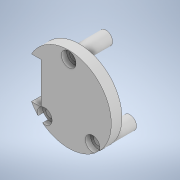
# Autodesk Inventor part: Driveunit_Spacer
Saved by Autodesk Inventor 2021 (Build 250183000, 183)
## iProperties
Created: 2024-08-04
Part Number: Driveunit_Spacer
Material: Generic
Document SubType Name: Modeling
Designer: Lukas
Density: 1 g/cm^3
Appearance: Default
Author: Lukas
Autodesk Inventor part; units mm, degrees
ref_plane "YZ Plane" through (0, 0, 0) normal (1, 0, 0) x (0, 1, 0)
ref_plane "XZ Plane" through (0, 0, 0) normal (0, 1, 0) x (-1, 0, 0)
ref_plane "XY Plane" through (0, 0, 0) normal (0, 0, 1) x (1, 0, 0)
sketch "Sketch1" plane through (0, 0, 0) normal (0, 0, 1) x (1, 0, 0)
  circle A0 centre (0, 0) radius 16
  line L0 (-16, 7.75) -> (-10.3, 7.75)
  line L1 (-10.3, 7.75) -> (-10.3, -7.75)
  line L2 (-10.3, -7.75) -> (-16, -7.75)
  line L3 (-16, -7.75) -> (-16, 7.75)
  circle A1 centre (-9, -10) radius 1.6
  circle A2 centre (9, -10) radius 1.6
  circle A3 centre (0, 13) radius 1.6
  circle A4 centre (0, 13) radius 2.5
  circle A5 centre (-9, -10) radius 2.5
  circle A6 centre (9, -10) radius 2.5
  point P0 (-10.3, 0)
  point P1 (-13.9978, -7.75)
  point P2 (-13.9978, 7.75)
  dimension "d0" = 32
  dimension "d1" = 5.7
  dimension "d2" = 15.5
  dimension "d3" = 9
  dimension "d4" = 9
  dimension "d5" = 23
  dimension "d6" = 13
  dimension "d7" = 3.2
  dimension "d8" = 5
  constraints: 8 end point, 7 centre point, 4 coincident, 4 equal radius, 2 horizontal alignment, 2 parallel, 1 horizontal, 1 midpoint, 1 perpendicular, 1 tangent, 1 vertical alignment
  measures "d0" diameter of A0
  measures "d1" distance of L0.start L0.end
  measures "d2" distance of L2.end L0.start
  measures "d3" horizontal distance of point (0, 0) A1.centre
  measures "d4" horizontal distance of A2.centre point (0, 0)
  measures "d5" vertical distance of A3.centre A1.centre
  measures "d6" distance of point (0, 0) A3.centre
  measures "d7" diameter of A3
  measures "d8" diameter of A5
extrude "Extrusion1" add sketch "Sketch1" along normal blind 4 contours A0 L2 L1 L0 | A4 | A5 | A6 picked at (0.1004, -2.0554)
extrude "Extrusion2" add sketch "Sketch1" against normal blind 10 contours A4 | A5 | A6
sketch "Sketch2" plane through (0, 0, 4) normal (0, 0, 1) x (1, 0, 0)
  circle A0 centre (0, 13) radius 1.6 projected
  circle A1 centre (-9, -10) radius 1.6 projected
  circle A2 centre (9, -10) radius 1.6 projected
  circle A3 centre (0, 13) radius 2.75
  circle A4 centre (-9, -10) radius 2.75
  circle A5 centre (9, -10) radius 2.75
  point P0 (0, 0)
  dimension "d14" = 5.5
  constraints: 3 centre point, 3 coincident, 2 equal radius
  measures "d14" diameter of A3
extrude "Extrusion3" cut sketch "Sketch2" against normal blind 2
equation "\"d4\" = d3"
body "Solid1"
